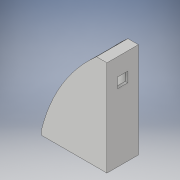
# Autodesk Inventor part: Pi Chassis
Saved by Autodesk Inventor 2017 (Build 210142000, 142)
## iProperties
Created: 2018-04-23
Part Number: Pi Chassis
Material: Generic
Document SubType Name: Modeling
Designer: student
Density: 1 g/cm^3
Appearance: Default
Author: student
Autodesk Inventor part; units mm, degrees
ref_plane "YZ Plane" through (0, 0, 0) normal (1, 0, 0) x (0, 1, 0)
ref_plane "XZ Plane" through (0, 0, 0) normal (0, 1, 0) x (-1, 0, 0)
ref_plane "XY Plane" through (0, 0, 0) normal (0, 0, 1) x (1, 0, 0)
sketch "Sketch1" plane through (0, 0, 0) normal (0, 0, 1) x (1, 0, 0)
  line L0 (0, 0) -> (82.55, 0)
  line L1 (82.55, 0) -> (82.55, 123.825)
  line L2 (82.55, 123.825) -> (0, 123.825)
  line L3 (0, 123.825) -> (0, 0)
  arc A0 (73.025, 123.825) -> (0, 6.35) centre (216.4664, -46.7758) ccw
  point P0 (60.325, 123.825)
  dimension "d0" = 82.55
  dimension "d1" = 123.825
  dimension "d5" = 9.525
  dimension "d6" = 6.35
  constraints: 8 end point, 3 point on line, 2 parallel, 2 point on circle, 1 centre point, 1 horizontal, 1 perpendicular
  measures "d0" distance of L2.end L1.end
  measures "d1" distance of L1.end L0.end
  measures "d5" distance from line of L1 A0.start
  measures "d6" distance from line of L0 A0.end
extrude "Extrusion1" add sketch "Sketch1" along normal mid plane 46.0375 contours L3 A0 L2 L1 L0
sketch "Sketch3" plane through (0, 0, 23.0187) normal (-1, 0, 0) x (0, 0, 1)
  line L0 (-39.6875, 117.475) -> (-6.35, 117.475)
  line L1 (-6.35, 117.475) -> (-6.35, 3.175)
  line L2 (-6.35, 3.175) -> (-39.6875, 3.175)
  line L3 (-39.6875, 3.175) -> (-39.6875, 117.475)
  line L4 (0, 6.35) -> (0, 123.825) projected
  line L5 (-46.0375, 123.825) -> (0, 123.825) projected
  point P0 (-23.0187, 0)
  dimension "d9" = 33.3375
  dimension "d10" = 114.3
  dimension "d11" = 6.35
  dimension "d12" = 6.35
  constraints: 8 end point, 2 parallel, 1 horizontal, 1 perpendicular
  measures "d9" distance of L1.end L2.end
  measures "d10" distance of L0.end L1.end
  measures "d11" distance between parallel lines of L4 L1
  measures "d12" distance between parallel lines of L5 L0
extrude "Extrusion2" cut sketch "Sketch3" along normal mid plane 158.75
sketch "Sketch4" plane through (79.375, 0, 23.0187) normal (-1, 0, 0) x (0, 0, 1)
  line L0 (-39.6875, 117.475) -> (-6.35, 117.475) projected
  line L1 (-39.6875, 117.475) -> (-6.35, 117.475) projected
  line L2 (-23.0188, 117.475) -> (-23.0188, 92.075)
  line L3 (-29.3688, 98.425) -> (-16.6688, 98.425)
  line L4 (-16.6688, 98.425) -> (-16.6688, 85.725)
  line L5 (-16.6688, 85.725) -> (-29.3688, 85.725)
  line L6 (-29.3688, 85.725) -> (-29.3688, 98.425)
  line L7 (-29.3688, 98.425) -> (-16.6688, 85.725) construction
  line L8 (-16.6688, 98.425) -> (-29.3688, 85.725) construction
  point P0 (-23.0187, 0)
  dimension "d26" = 25.4
  dimension "d27" = 12.7
  dimension "d28" = 12.7
  constraints: 14 end point, 3 midpoint, 2 parallel, 1 horizontal, 1 perpendicular, 1 vertical
  measures "d26" distance of L2.start L2.end
  measures "d27" distance of L4.end L5.end
  measures "d28" distance of L3.end L4.end
extrude "Extrusion3" cut sketch "Sketch4" against normal through all
sketch "Sketch5" plane through (0, 3.175, 16.6688) normal (0, 1, 0) x (1, 0, 0)
  line L0 (60.325, 26.9875) -> (22.225, 26.9875)
  line L1 (22.225, 26.9875) -> (22.225, 3.175)
  line L2 (22.225, 3.175) -> (60.325, 3.175)
  line L3 (60.325, 3.175) -> (60.325, 26.9875)
  line L4 (65.7954, 33.3375) -> (0, 33.3375) projected
  line L5 (0, 0) -> (65.7954, 0) projected
  line L6 (0, 0) -> (0, 33.3375) projected
  point P0 (0, 16.6688)
  dimension "d20" = 6.35
  dimension "d21" = 3.175
  dimension "d22" = 22.225
  dimension "d23" = 38.1
  constraints: 8 end point, 2 parallel, 1 horizontal, 1 perpendicular
  measures "d20" distance between parallel lines of L4 L0
  measures "d21" distance between parallel lines of L5 L2
  measures "d22" distance between parallel lines of L6 L1
  measures "d23" distance of L0.start L0.end
extrude "Extrusion4" cut sketch "Sketch5" against normal blind 63.5
sketch "Sketch6" plane through (73.025, 123.825, 23.0187) normal (0, 1, 0) x (1, 0, 0)
  line L0 (9.525, 46.0375) -> (9.525, 0) projected
  line L1 (-73.025, 0) -> (9.525, 0) projected
  line L2 (9.525, 46.0375) -> (-7.684, 46.0375)
  line L3 (-7.684, 46.0375) -> (-7.684, 0)
  line L4 (-7.684, 0) -> (9.525, 0)
  line L5 (9.525, 0) -> (9.525, 46.0375)
  point P0 (-73.025, 23.0187)
  constraints: 8 end point, 2 parallel, 1 horizontal, 1 perpendicular, 1 point on line
extrude "Extrusion5" cut sketch "Sketch6" against normal blind 3.175
sketch "Sketch7" plane through (0, 0, 23.0187) normal (0, 0, 1) x (1, 0, 0)
  line L0 (82.55, 120.65) -> (82.55, 0) projected
  line L1 (0, 0) -> (82.55, 0)
  line L2 (82.55, 0) -> (82.55, 120.65)
  line L3 (82.55, 120.65) -> (0, 120.65)
  line L4 (0, 120.65) -> (0, 0)
  constraints: 8 end point, 2 parallel, 1 horizontal, 1 perpendicular
extrude "Extrusion6" cut sketch "Sketch7" against normal blind 3.175
sketch "Sketch8" plane through (0, 0, -23.0187) normal (0, 0, -1) x (-1, 0, 0)
  line L0 (0, 0) -> (0, 6.35) projected
  line L1 (-82.55, 120.65) -> (-82.55, 0) projected
  line L2 (0, 0) -> (-82.55, 0)
  line L3 (-82.55, 0) -> (-82.55, 120.65)
  line L4 (-82.55, 120.65) -> (0, 120.65)
  line L5 (0, 120.65) -> (0, 0)
  constraints: 8 end point, 2 parallel, 1 horizontal, 1 perpendicular
extrude "Extrusion7" cut sketch "Sketch8" against normal blind 3.175
body "Solid1"
